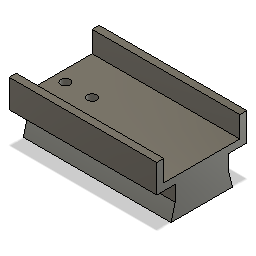
PST to dovetail (Autodesk Fusion 360 design; units mm, degrees)
Autodesk Fusion 360 part; units mm, degrees
note: some values were not read from the file. Set by a fixed rule: which sketch regions a step uses.
sketch "Sketch1" plane through (0, 0, 0) normal (1, 0, 0) x (0, 0, -1)
  line L0 (0, 0) -> (27, 0)
  line L1 (0, 0) -> (0, 15)
  line L2 (0, 15) -> (-5, 15)
  line L3 (-5, 15) -> (-5, -5)
  line L4 (27, -27) -> (5.0925, -27)
  line L5 (-5, -5) -> (8.0399, -5)
  line L6 (27, 0) -> (27, -27) construction
  line L7 (27, -27) -> (48.9075, -27)
  line L8 (59, -5) -> (45.9601, -5)
  line L9 (54, 0) -> (27, 0)
  line L10 (54, 0) -> (54, 15)
  line L11 (54, 15) -> (59, 15)
  line L12 (59, 15) -> (59, -5)
  line L13 (5.0925, -27) -> (14.9145, -27) construction
  line L14 (8.0399, -5) -> (8.0399, -16)
  line L15 (8.0399, -16) -> (5.0925, -27)
  line L16 (45.9601, -5) -> (45.9601, -16)
  line L17 (45.9601, -16) -> (48.9075, -27)
  dimension "d5" = 15
  dimension "d28" = 21.9075
  dimension "d30" = 5
  dimension "d33" = 27
  dimension "d41" = 5
  dimension "d49" = 11
  dimension "d50" = 75
  dimension "d51" = 11
  constraint coincident L0.start L1.start
  constraint horizontal L5
  constraint perpendicular L3 L5
  constraint parallel L1 L3
  constraint perpendicular L4 L6
  constraint parallel L0 L4
  constraint parallel L1 L6
  constraint parallel L2 L5
  constraint symmetric L0.start L6 L9.start
  constraint symmetric L3.end L6 L8.start
  constraint symmetric L1.end L6 L10.end
  constraint symmetric L2.end L6 L11.end
  constraint symmetric L5.end L6 L8.end
  constraint symmetric L4.end L6 L7.end
  constraint symmetric L0.end L6 L9.end
  constraint symmetric L4.start L6 L7.start
  constraint horizontal L13
  constraint perpendicular L5 L14
  constraint symmetric L6 L14.end L16.end
  measures "d5" distance of L0.start L1.end
  measures "d28" distance of L4.end L4.start
  measures "d30" distance of L1 L3
  measures "d33" distance of L1 L6
  measures "d41" distance of L0.start L5
  measures "d49" distance of L4 L14.end
  measures "d50" angle of L13 L15
  measures "d51" distance of L5.end L14.end
extrude "Extrude1" add sketch "Sketch1" along normal blind 35
sketch "Sketch2" plane through (0, -27, 0) normal (0, -1, 0) x (1, 0, 0)
  line L0 (0, -5.0925) -> (0, -48.9075)
  line L1 (35, -48.9075) -> (35, -5.0925)
  circle A0 centre (8, -27) radius 3.3
  circle A1 centre (8, -27) radius 5.75
  line L2 (17.5, -5.6) -> (17.5, -37) construction
  circle A2 centre (27, -27) radius 5.75
  circle A3 centre (27, -27) radius 3.3
  line L3 (0, -27) -> (17.5, -27)
  line L4 (0, -48.9075) -> (35, -48.9075)
  line L5 (35, -5.0925) -> (0, -5.0925)
  dimension "d20" = 6.6
  dimension "d23" = 11.5
  dimension "d36" = 9.5
  constraint concentric A0 A1
  constraint symmetric A0 L2 A3
  constraint symmetric A1 L2 A2
  constraint midpoint L0 L3.start
  constraint coincident L2 L3.end
  constraint perpendicular L2 L3
  measures "d20" diameter of A0
  measures "d23" diameter of A1
  measures "d36" distance of A0.centre L2
extrude "Extrude2" cut sketch "Sketch2" against normal up to surface (27 mm away) contours A0 L3 | A0 L3 | A3
extrude "Extrude3" cut sketch "Sketch2" against normal up to surface (10 mm away) contours A0 A1 L3 | A0 A1 L3 | A2
extrude "Extrude4" add 1 faces at (35, -23.3333, -20.68) along direction (1, 0, 0) blind 70
equation "d28 = 1.725 in / 2"
equation "d36 = ( 19 / 2 ) * 1 mm"
